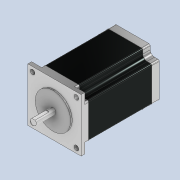
# Autodesk Inventor part: Nema 23 Dual Shaft 87mm Stepper Motor
Saved by Autodesk Inventor 2022 (Build 260153000, 153)
## iProperties
Created: 2021-10-10
Part Number: Nema 23 Dual Shaft 87mm Stepper Motor
Material: Generic
Document SubType Name: Modeling
Designer: Coy
Density: 1 g/cm^3
Appearance: Default
Author: Coy
Autodesk Inventor part; units mm, degrees
ref_plane "YZ Plane" through (0, 0, 0) normal (1, 0, 0) x (0, 1, 0)
ref_plane "XZ Plane" through (0, 0, 0) normal (0, 1, 0) x (-1, 0, 0)
ref_plane "XY Plane" through (0, 0, 0) normal (0, 0, 1) x (1, 0, 0)
sketch "Sketch1" plane through (0, 0, 0) normal (0, 0, 1) x (1, 0, 0)
  line L0 (0, 0) -> (57.3, 0)
  line L1 (57.3, 0) -> (57.3, 57.3)
  line L2 (57.3, 57.3) -> (0, 57.3)
  line L3 (0, 57.3) -> (0, 0)
  line L4 (5.08, 52.22) -> (52.22, 52.22) construction
  line L5 (52.22, 52.22) -> (52.22, 5.08) construction
  line L6 (52.22, 5.08) -> (5.08, 5.08) construction
  line L7 (5.08, 5.08) -> (5.08, 52.22) construction
  line L8 (5.08, 52.22) -> (5.08, 57.3) construction
  line L9 (5.08, 52.22) -> (0, 52.22) construction
  line L10 (52.22, 5.08) -> (52.22, 0) construction
  line L11 (52.22, 5.08) -> (57.3, 5.08) construction
  circle A0 centre (5.08, 52.22) radius 2.55
  circle A1 centre (52.22, 52.22) radius 2.55
  circle A2 centre (5.08, 5.08) radius 2.55
  circle A3 centre (52.22, 5.08) radius 2.55
  line L12 (28.65, 57.3) -> (28.65, 0) construction
  circle A4 centre (28.65, 28.65) radius 19.55
  dimension "d0" = 57.3
  dimension "d1" = 57.3
  dimension "d2" = 47.14
  dimension "d3" = 47.14
  dimension "d4" = 5.1
  dimension "d5" = 5.1
  dimension "d6" = 5.1
  dimension "d7" = 5.1
  dimension "d8" = 39.1
  constraints: 26 end point, 6 parallel, 6 perpendicular, 5 centre point, 4 coincident, 4 point on line, 3 midpoint, 2 horizontal
  measures "d0" distance of L2.end L1.end
  measures "d1" distance of L1.end L0.end
  measures "d2" distance of L5.end L6.end
  measures "d3" distance of L4.end L5.end
  measures "d4" diameter of A0
  measures "d5" diameter of A1
  measures "d6" diameter of A2
  measures "d7" diameter of A3
  measures "d8" diameter of A4
extrude "Extrusion1" add sketch "Sketch1" against normal blind 4 contours L3 L2 L1 L0 | A4
sketch "Sketch2" plane through (0, 0, 0) normal (0, 0, 1) x (1, 0, 0)
  line L0 (0, 57.3) -> (57.3, 57.3) construction
  line L1 (28.65, 57.3) -> (28.65, 0) construction
  line L2 (57.3, 0) -> (0, 0) construction
  circle A0 centre (28.65, 28.65) radius 19.05
  dimension "d11" = 38.1
  constraints: 3 midpoint, 2 end point, 1 centre point
  measures "d11" diameter of A0
extrude "Extrusion2" add sketch "Sketch2" along normal blind 1.6
sketch "Sketch3" plane through (28.65, 28.65, 1.6) normal (0, 0, 1) x (1, 0, 0)
  circle A0 centre (0, 0) radius 3.175
  point P0 (-28.65, -28.65)
  dimension "d14" = 6.35
  constraints: 1 centre point
  measures "d14" diameter of A0
extrude "Extrusion3" add sketch "Sketch3" along normal blind 21
sketch "Sketch4" plane through (28.65, 28.65, 22.6) normal (0, 0, 1) x (1, 0, 0)
  circle A0 centre (0, 0) radius 3.175 projected
  line L0 (-1.7103, 2.675) -> (1.7103, 2.675)
  point P0 (-28.65, -28.65)
  dimension "d17" = 2.675
  constraints: 2 end point, 2 point on circle, 1 horizontal
  measures "d17" distance from line of A0.centre L0
extrude "Extrusion4" cut sketch "Sketch4" against normal blind 15 contours L0 A0 picked at (-0.3543, 2.7806)
sketch "Sketch5" plane through (0, 0, -4) normal (0, 0, -1) x (-1, 0, 0)
  line L0 (-57.3, 57.3) -> (-57.3, 0) projected
  line L1 (-57.3, 0) -> (0, 0) projected
  line L2 (0, 0) -> (0, 57.3) projected
  line L3 (0, 57.3) -> (-57.3, 57.3) projected
  circle A0 centre (-5.08, 52.22) radius 2.55 projected
  circle A1 centre (-52.22, 52.22) radius 2.55 projected
  circle A2 centre (-5.08, 5.08) radius 2.55 projected
  circle A3 centre (-52.22, 5.08) radius 2.55 projected
  arc A4 (-52.22, 47.67) -> (-47.67, 52.22) centre (-52.22, 52.22) ccw
  arc A5 (-9.63, 52.22) -> (-5.08, 47.67) centre (-5.08, 52.22) ccw
  arc A6 (-5.08, 9.63) -> (-9.63, 5.08) centre (-5.08, 5.08) ccw
  arc A7 (-47.67, 5.08) -> (-52.22, 9.63) centre (-52.22, 5.08) ccw
  line L4 (0, 57.3) -> (-57.3, 57.3) projected
  line L5 (-47.67, 55.8) -> (-47.67, 52.22)
  line L6 (-9.63, 55.8) -> (-9.63, 52.22)
  line L7 (-57.3, 0) -> (-57.3, 57.3) projected
  line L8 (-55.8, 47.67) -> (-52.22, 47.67)
  line L9 (-55.8, 9.63) -> (-52.22, 9.63)
  line L10 (0, 0) -> (-57.3, 0) projected
  line L11 (-47.67, 1.5) -> (-47.67, 5.08)
  line L12 (-9.63, 1.5) -> (-9.63, 5.08)
  line L13 (0, 57.3) -> (0, 0) projected
  line L14 (-1.5, 47.67) -> (-5.08, 47.67)
  line L15 (-1.5, 9.63) -> (-5.08, 9.63)
  line L16 (0, 0) -> (0, 57.3) projected
  line L17 (-57.3, 0) -> (0, 0) projected
  line L18 (-57.3, 57.3) -> (-57.3, 0) projected
  arc A8 (-55.8, 47.67) -> (-57.3, 46.17) centre (-55.8, 46.17) ccw
  arc A9 (-46.17, 57.3) -> (-47.67, 55.8) centre (-46.17, 55.8) ccw
  arc A10 (-9.63, 55.8) -> (-11.13, 57.3) centre (-11.13, 55.8) ccw
  arc A11 (0, 46.17) -> (-1.5, 47.67) centre (-1.5, 46.17) ccw
  arc A12 (-1.5, 9.63) -> (0, 11.13) centre (-1.5, 11.13) ccw
  arc A13 (-11.13, 0) -> (-9.63, 1.5) centre (-11.13, 1.5) ccw
  arc A14 (-47.67, 1.5) -> (-46.17, 0) centre (-46.17, 1.5) ccw
  arc A15 (-57.3, 11.13) -> (-55.8, 9.63) centre (-55.8, 11.13) ccw
  dimension "d20" = 2
  dimension "d21" = 2
  dimension "d22" = 2
  dimension "d23" = 2
  dimension "d24" = 3
  dimension "d25" = 3
  dimension "d26" = 3
  dimension "d27" = 3
  dimension "d28" = 3
  dimension "d29" = 3
  dimension "d30" = 3
  dimension "d31" = 3
  constraints: 24 point on circle, 18 tangent, 16 end point, 12 centre point, 4 horizontal, 3 point on line, 2 perpendicular, 2 vertical, 14 other
  measures "d20" radial gap between concentric circles of A1 A4
  measures "d21" radial gap between concentric circles of A0 A5
  measures "d22" radial gap between concentric circles of A2 A6
  measures "d23" radial gap between concentric circles of A3 A7
  measures "d24" diameter of A8
  measures "d25" diameter of A9
  measures "d26" diameter of A10
  measures "d27" diameter of A11
  measures "d28" diameter of A12
  measures "d29" diameter of A13
  measures "d30" diameter of A14
  measures "d31" diameter of A15
extrude "Extrusion5" add sketch "Sketch5" along normal blind 4 contours A8 L8 A4 L5 A9 L3 A10 L6 A5 L14 A11 L2 A12 L15 A6 L12 A13 L1 A14 L11 A7 L9 A15 L0
sketch "Sketch6" plane through (0, 0, -8) normal (0, 0, -1) x (-1, 0, 0)
  arc A0 (-52.22, 47.67) -> (-47.67, 52.22) centre (-52.22, 52.22) ccw projected
  line L0 (-52.22, 47.67) -> (-55.8, 47.67) projected
  arc A1 (-55.8, 47.67) -> (-57.3, 46.17) centre (-55.8, 46.17) ccw projected
  line L1 (-57.3, 46.17) -> (-57.3, 11.13) projected
  arc A2 (-57.3, 11.13) -> (-55.8, 9.63) centre (-55.8, 11.13) ccw projected
  line L2 (-55.8, 9.63) -> (-52.22, 9.63) projected
  arc A3 (-47.67, 5.08) -> (-52.22, 9.63) centre (-52.22, 5.08) ccw projected
  line L3 (-47.67, 5.08) -> (-47.67, 1.5) projected
  arc A4 (-47.67, 1.5) -> (-46.17, 0) centre (-46.17, 1.5) ccw projected
  line L4 (-46.17, 0) -> (-11.13, 0) projected
  arc A5 (-11.13, 0) -> (-9.63, 1.5) centre (-11.13, 1.5) ccw projected
  line L5 (-9.63, 1.5) -> (-9.63, 5.08) projected
  arc A6 (-5.08, 9.63) -> (-9.63, 5.08) centre (-5.08, 5.08) ccw projected
  line L6 (-5.08, 9.63) -> (-1.5, 9.63) projected
  arc A7 (-1.5, 9.63) -> (0, 11.13) centre (-1.5, 11.13) ccw projected
  line L7 (0, 11.13) -> (0, 46.17) projected
  arc A8 (0, 46.17) -> (-1.5, 47.67) centre (-1.5, 46.17) ccw projected
  line L8 (-1.5, 47.67) -> (-5.08, 47.67) projected
  arc A9 (-9.63, 52.22) -> (-5.08, 47.67) centre (-5.08, 52.22) ccw projected
  line L9 (-9.63, 52.22) -> (-9.63, 55.8) projected
  arc A10 (-9.63, 55.8) -> (-11.13, 57.3) centre (-11.13, 55.8) ccw projected
  line L10 (-11.13, 57.3) -> (-46.17, 57.3) projected
  arc A11 (-46.17, 57.3) -> (-47.67, 55.8) centre (-46.17, 55.8) ccw projected
  line L11 (-47.67, 55.8) -> (-47.67, 52.22) projected
  line L12 (-55.8, 47.47) -> (-52.22, 47.47)
  arc A12 (-52.22, 47.47) -> (-47.47, 52.22) centre (-52.22, 52.22) ccw
  line L13 (-47.47, 52.22) -> (-47.47, 55.8)
  arc A13 (-46.17, 57.1) -> (-47.47, 55.8) centre (-46.17, 55.8) ccw
  line L14 (-46.17, 57.1) -> (-11.13, 57.1)
  arc A14 (-9.83, 55.8) -> (-11.13, 57.1) centre (-11.13, 55.8) ccw
  line L15 (-9.83, 55.8) -> (-9.83, 52.22)
  arc A15 (-9.83, 52.22) -> (-5.08, 47.47) centre (-5.08, 52.22) ccw
  line L16 (-5.08, 47.47) -> (-1.5, 47.47)
  arc A16 (-0.2, 46.17) -> (-1.5, 47.47) centre (-1.5, 46.17) ccw
  line L17 (-0.2, 46.17) -> (-0.2, 11.13)
  arc A17 (-1.5, 9.83) -> (-0.2, 11.13) centre (-1.5, 11.13) ccw
  line L18 (-1.5, 9.83) -> (-5.08, 9.83)
  arc A18 (-5.08, 9.83) -> (-9.83, 5.08) centre (-5.08, 5.08) ccw
  line L19 (-9.83, 5.08) -> (-9.83, 1.5)
  arc A19 (-11.13, 0.2) -> (-9.83, 1.5) centre (-11.13, 1.5) ccw
  line L20 (-11.13, 0.2) -> (-46.17, 0.2)
  arc A20 (-47.47, 1.5) -> (-46.17, 0.2) centre (-46.17, 1.5) ccw
  line L21 (-47.47, 1.5) -> (-47.47, 5.08)
  arc A21 (-47.47, 5.08) -> (-52.22, 9.83) centre (-52.22, 5.08) ccw
  line L22 (-52.22, 9.83) -> (-55.8, 9.83)
  arc A22 (-57.1, 11.13) -> (-55.8, 9.83) centre (-55.8, 11.13) ccw
  line L23 (-57.1, 11.13) -> (-57.1, 46.17)
  arc A23 (-55.8, 47.47) -> (-57.1, 46.17) centre (-55.8, 46.17) ccw
  point P0 (0, 0)
  dimension "d34" = 0.2
  constraints: 24 end point, 24 point on circle, 12 centre point, 23 other
  measures "d34" distance between parallel lines of L0 L12
extrude "Extrusion6" add sketch "Sketch6" along normal blind 68 contours L12 A12 L13 A13 L14 A14 L15 A15 L16 A16 L17 A17 L18 A18 L19 A19 L20 A20 L21 A21 L22 A22 L23 A23
sketch "Sketch7" plane through (0, 0, -76) normal (0, 0, -1) x (-1, 0, 0)
  arc A0 (-57.1, 11.13) -> (-55.8, 9.83) centre (-55.8, 11.13) ccw projected
  line L0 (-57.1, 11.13) -> (-57.1, 46.17) projected
  arc A1 (-55.8, 47.47) -> (-57.1, 46.17) centre (-55.8, 46.17) ccw projected
  line L1 (-55.8, 47.47) -> (-52.22, 47.47) projected
  arc A2 (-52.22, 47.47) -> (-47.47, 52.22) centre (-52.22, 52.22) ccw projected
  line L2 (-47.47, 52.22) -> (-47.47, 55.8) projected
  arc A3 (-46.17, 57.1) -> (-47.47, 55.8) centre (-46.17, 55.8) ccw projected
  line L3 (-46.17, 57.1) -> (-11.13, 57.1) projected
  arc A4 (-9.83, 55.8) -> (-11.13, 57.1) centre (-11.13, 55.8) ccw projected
  line L4 (-9.83, 55.8) -> (-9.83, 52.22) projected
  arc A5 (-9.83, 52.22) -> (-5.08, 47.47) centre (-5.08, 52.22) ccw projected
  line L5 (-5.08, 47.47) -> (-1.5, 47.47) projected
  arc A6 (-0.2, 46.17) -> (-1.5, 47.47) centre (-1.5, 46.17) ccw projected
  line L6 (-0.2, 46.17) -> (-0.2, 11.13) projected
  arc A7 (-1.5, 9.83) -> (-0.2, 11.13) centre (-1.5, 11.13) ccw projected
  line L7 (-1.5, 9.83) -> (-5.08, 9.83) projected
  arc A8 (-5.08, 9.83) -> (-9.83, 5.08) centre (-5.08, 5.08) ccw projected
  line L8 (-9.83, 5.08) -> (-9.83, 1.5) projected
  arc A9 (-11.13, 0.2) -> (-9.83, 1.5) centre (-11.13, 1.5) ccw projected
  line L9 (-11.13, 0.2) -> (-46.17, 0.2) projected
  arc A10 (-47.47, 1.5) -> (-46.17, 0.2) centre (-46.17, 1.5) ccw projected
  line L10 (-47.47, 1.5) -> (-47.47, 5.08) projected
  arc A11 (-47.47, 5.08) -> (-52.22, 9.83) centre (-52.22, 5.08) ccw projected
  line L11 (-52.22, 9.83) -> (-55.8, 9.83) projected
  arc A12 (-52.22, 47.67) -> (-47.67, 52.22) centre (-52.22, 52.22) ccw projected
  line L12 (-52.22, 47.67) -> (-55.8, 47.67) projected
  arc A13 (-55.8, 47.67) -> (-57.3, 46.17) centre (-55.8, 46.17) ccw projected
  line L13 (-57.3, 46.17) -> (-57.3, 11.13) projected
  arc A14 (-57.3, 11.13) -> (-55.8, 9.63) centre (-55.8, 11.13) ccw projected
  line L14 (-55.8, 9.63) -> (-52.22, 9.63) projected
  arc A15 (-47.67, 5.08) -> (-52.22, 9.63) centre (-52.22, 5.08) ccw projected
  line L15 (-47.67, 5.08) -> (-47.67, 1.5) projected
  arc A16 (-47.67, 1.5) -> (-46.17, 0) centre (-46.17, 1.5) ccw projected
  line L16 (-46.17, 0) -> (-11.13, 0) projected
  arc A17 (-11.13, 0) -> (-9.63, 1.5) centre (-11.13, 1.5) ccw projected
  line L17 (-9.63, 1.5) -> (-9.63, 5.08) projected
  arc A18 (-5.08, 9.63) -> (-9.63, 5.08) centre (-5.08, 5.08) ccw projected
  line L18 (-5.08, 9.63) -> (-1.5, 9.63) projected
  arc A19 (-1.5, 9.63) -> (0, 11.13) centre (-1.5, 11.13) ccw projected
  line L19 (0, 11.13) -> (0, 46.17) projected
  arc A20 (0, 46.17) -> (-1.5, 47.67) centre (-1.5, 46.17) ccw projected
  line L20 (-1.5, 47.67) -> (-5.08, 47.67) projected
  arc A21 (-9.63, 52.22) -> (-5.08, 47.67) centre (-5.08, 52.22) ccw projected
  line L21 (-9.63, 52.22) -> (-9.63, 55.8) projected
  arc A22 (-9.63, 55.8) -> (-11.13, 57.3) centre (-11.13, 55.8) ccw projected
  line L22 (-11.13, 57.3) -> (-46.17, 57.3) projected
  arc A23 (-46.17, 57.3) -> (-47.67, 55.8) centre (-46.17, 55.8) ccw projected
  line L23 (-47.67, 55.8) -> (-47.67, 52.22) projected
  point P0 (0, 0)
extrude "Extrusion7" add sketch "Sketch7" along normal blind 8 contours L0 A1 L1 A2 L2 A3 L3 A4 L4 A5 L5 A6 L6 A7 L7 A8 L8 A9 L9 A10 L10 A11 L11 A0 | A12 L23 A23 L22 A22 L21 A21 L20 A20 L19 A19 L18 A18 L17 A17 L16 A16 L15 A15 L14 A14 L13 A13 L12
sketch "Sketch8" plane through (0, 0, -84) normal (0, 0, -1) x (-1, 0, 0)
  line L0 (-46.17, 0) -> (-11.13, 0) construction
  line L1 (-28.65, 0) -> (-28.65, 57.1) construction
  line L2 (-46.17, 57.1) -> (-11.13, 57.1) construction
  arc A0 (-30.3603, 31.325) -> (-26.9397, 31.325) centre (-28.65, 28.65) ccw projected
  circle A1 centre (-28.65, 28.65) radius 3.175
  point P0 (0, 0)
  dimension "d39" = 6.35
  constraints: 2 end point, 2 midpoint, 1 centre point, 1 coincident
  measures "d39" diameter of A1
extrude "Extrusion8" add sketch "Sketch8" along normal blind 15
sketch "Sketch9" plane through (11.13, 0, -76) normal (0, -1, 0) x (1, 0, 0)
  line L0 (0, -8) -> (35.04, -8) projected
  line L1 (0, 0) -> (35.04, 0) projected
  line L2 (13.52, -8) -> (21.52, -8)
  line L3 (21.52, -8) -> (21.52, 0)
  line L4 (21.52, 0) -> (13.52, 0)
  line L5 (13.52, 0) -> (13.52, -8)
  line L6 (14.345, -23) -> (20.695, -23) construction
  line L7 (17.52, -23) -> (17.52, 8.4393) construction
  line L8 (17.52, 0) -> (17.52, -8) construction
  point P0 (-11.13, 76)
  point P1 (13.52, 0)
  point P2 (21.52, -8)
  dimension "d42" = 8
  dimension "d43" = 0
  constraints: 12 end point, 3 midpoint, 2 parallel, 2 point on line, 1 horizontal, 1 perpendicular, 1 vertical
  measures "d42" distance of L4.end L3.end
  measures "d43" distance between parallel lines of L7 L8
extrude "Extrusion9" add sketch "Sketch9" along normal blind 1
equation "\"d5\" = d4"
equation "\"d6\" = d4"
equation "\"d7\" = d4"
equation "\"d25\" = d24"
equation "\"d26\" = d24"
equation "\"d27\" = d24"
equation "\"d28\" = d24"
equation "\"d29\" = d24"
equation "\"d30\" = d24"
equation "\"d31\" = d24"
body "Solid1"
